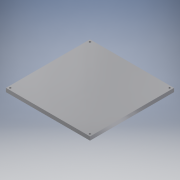
# Autodesk Inventor part: Byggeplade
Saved by Autodesk Inventor 2016 SP1 (Build 200210100, 210)
## iProperties
Created: 2015-05-11
Part Number: Byggeplade
Material: Aluminum 6061
Document SubType Name: Modeling
Designer: Mathias Lyngklip Kjeldgaard
Density: 2.71 g/cm^3
Appearance: Aluminum - Flat
Mass: 1431.46 g
Surface Area: 1154.71 cm^2
Volume: 528.215 cm^3
Author: Mathias Lyngklip Kjeldgaard
Autodesk Inventor part; units mm, degrees
ref_plane "YZ Plane" through (0, 0, 0) normal (1, 0, 0) x (0, 1, 0)
ref_plane "XZ Plane" through (0, 0, 0) normal (0, 1, 0) x (-1, 0, 0)
ref_plane "XY Plane" through (0, 0, 0) normal (0, 0, 1) x (1, 0, 0)
sketch "Sketch1" plane through (0, 0, 0) normal (0, 0, 1) x (1, 0, 0)
  line L0 (-115, 115) -> (115, 115)
  line L1 (115, 115) -> (115, -115)
  line L2 (115, -115) -> (-115, -115)
  line L3 (-115, -115) -> (-115, 115)
  point P0 (0, 0)
  dimension "d0" = 230
  dimension "d1" = 230
  dimension "d2" = 115
  dimension "d3" = 115
  constraints: 8 end point, 2 parallel, 1 horizontal, 1 perpendicular
  measures "d0" distance of L1.end L2.end
  measures "d1" distance of L0.end L1.end
  measures "d2" distance from line of point (0, 0) L0
  measures "d3" distance from line of point (0, 0) L1
extrude "Tykkelsen" add sketch "Sketch1" along normal blind 10
sketch "Sketch2" plane through (0, 0, 10) normal (0, 0, 1) x (1, 0, 0)
  line L0 (115, 115) -> (-115, 115) projected
  line L1 (-115, 115) -> (-115, -115) projected
  line L2 (-115, -115) -> (115, -115) projected
  line L3 (115, -115) -> (115, 115) projected
  circle A0 centre (109, -109) radius 2.5
  circle A1 centre (109, 109) radius 2.5
  circle A2 centre (-109, 109) radius 2.5
  circle A3 centre (-109, -109) radius 2.5
  point P0 (0, 0)
  dimension "d6" = 5
  dimension "d7" = 5
  dimension "d8" = 5
  dimension "d9" = 5
  dimension "d10" = 6
  dimension "d11" = 6
  dimension "d12" = 6
  dimension "d13" = 6
  dimension "d14" = 6
  dimension "d15" = 6
  dimension "d16" = 6
  dimension "d17" = 6
  dimension "d20" = 218
  dimension "d21" = 218
  constraints: 4 centre point
  measures "d6" diameter of A3
  measures "d7" diameter of A0
  measures "d8" diameter of A1
  measures "d9" diameter of A2
  measures "d10" distance from line of L3 A0.centre
  measures "d11" distance from line of L3 A1.centre
  measures "d12" distance from line of L2 A0.centre
  measures "d13" distance from line of L0 A1.centre
  measures "d14" distance from line of L2 A3.centre
  measures "d15" distance from line of L0 A2.centre
  measures "d16" distance from line of L1 A3.centre
  measures "d17" distance from line of L1 A2.centre
  measures "d20" distance of A0.centre A3.centre
  measures "d21" distance of A0.centre A1.centre
extrude "Monteringshuller" cut sketch "Sketch2" against normal blind 34.5 contours A0 | A1 | A2 | A3
equation "\"d2\" = 0.5 * d1"
equation "\"d3\" = 0.5 * d0"
equation "\"d6\" = d7"
equation "\"d8\" = d7"
equation "\"d9\" = d7"
equation "\"d11\" = d10"
equation "\"d13\" = d12"
equation "\"d14\" = d12"
equation "\"d15\" = d13"
equation "\"d16\" = d10"
equation "\"d17\" = d10"
body "Solid1"
